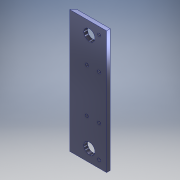
# Autodesk Inventor part: Ostrze
Saved by Autodesk Inventor 2017 (Build 210142000, 142)
## iProperties
Created: 2016-11-09
Part Number: Ostrze
Material: Generic
Document SubType Name: Modeling
Designer: Shichi
Density: 1 g/cm^3
Appearance: Chrome - Polished Blue
Author: Shichi
Autodesk Inventor part; units mm, degrees
ref_plane "YZ Plane" through (0, 0, 0) normal (1, 0, 0) x (0, 1, 0)
ref_plane "XZ Plane" through (0, 0, 0) normal (0, 1, 0) x (-1, 0, 0)
ref_plane "XY Plane" through (0, 0, 0) normal (0, 0, 1) x (1, 0, 0)
sketch "Sketch1" plane through (0, 0, 0) normal (0, 1, 0) x (-1, 0, 0)
  line L0 (0, 100) -> (-30, 100)
  line L1 (-30, 100) -> (-30, 0)
  line L2 (-30, 0) -> (0, 0)
  line L3 (0, 0) -> (0, 100)
  circle A0 centre (-24, 94) radius 1.25
  circle A1 centre (-24, 68) radius 1.25
  circle A2 centre (-14, 68) radius 1.25
  line L4 (-30, 50) -> (0, 50) construction
  circle A3 centre (-24, 6) radius 1.25
  circle A4 centre (-24, 32) radius 1.25
  circle A5 centre (-14, 32) radius 1.25
  circle A6 centre (-16, 90) radius 4.5
  circle A7 centre (-16, 10) radius 4.5
  dimension "d0" = 30
  dimension "d1" = 100
  dimension "d7" = 2.5
  dimension "d8" = 6
  dimension "d9" = 6
  dimension "d10" = 2.5
  dimension "d12" = 2.5
  dimension "d13" = 10
  dimension "d16" = 32
  dimension "d23" = 9
  dimension "d24" = 10
  dimension "d25" = 14
  constraints: 10 end point, 8 centre point, 4 symmetric about line, 2 midpoint, 2 parallel, 2 vertical alignment, 1 coincident, 1 horizontal, 1 horizontal alignment, 1 perpendicular, 4 other
  measures "d0" distance of L0.start L0.end
  measures "d1" distance of L0.end L1.end
  measures "d7" diameter of A0
  measures "d8" distance from line of A0.centre L1
  measures "d9" distance from line of L0 A0.centre
  measures "d10" diameter of A1
  measures "d12" diameter of A2
  measures "d13" distance of A2.centre A1.centre
  measures "d16" distance from line of L0 A2.centre
  measures "d23" diameter of A6
  measures "d24" distance from line of L0 A6.centre
  measures "d25" distance from line of L1 A6.centre
extrude "Extrusion1" add sketch "Sketch1" along normal blind 3 contours L3 L2 L1 L0 | A0 | A1 | A2 | A3 | A4 | A5 | A6 | A7
sketch "Sketch2" plane through (0, 0, 100) normal (0, 0, 1) x (1, 0, 0)
  line L0 (0, 0) -> (0, 3) projected
  line L1 (0, 0) -> (3, 3)
  line L2 (0, 3) -> (30, 3) projected
  line L3 (0, 3) -> (0, 0)
  dimension "d4" = 3
  constraints: 4 end point, 1 point on line, 1 vertical
  measures "d4" distance of L0.end L1.end
extrude "Extrusion2" cut sketch "Sketch2" against normal through all
extrude "Extrusion3" cut sketch "Sketch1" along normal through all contours A0 | A1 | A2 | A3 | A4 | A5
sketch "Sketch3" plane through (0, 3, 0) normal (0, 1, 0) x (1, 0, 0)
  circle A0 centre (16, -10) radius 4.5
  line L0 (3, 0) -> (3, -100) projected
  line L1 (30, 0) -> (3, 0) projected
  line L2 (3, -50) -> (16, -50) construction
  circle A1 centre (16, -90) radius 4.5
  line L3 (30, -100) -> (30, 0) projected
  point P0 (0, 0)
  dimension "d18" = 10
  dimension "d19" = 9
  dimension "d22" = 14
  constraints: 2 centre point, 2 end point, 1 horizontal, 1 midpoint, 1 symmetric about line, 1 other
  measures "d18" distance from line of L1 A0.centre
  measures "d19" diameter of A0
  measures "d22" distance from line of L3 A0.centre
extrude "Extrusion4" cut sketch "Sketch3" against normal through all
body "Solid1"
